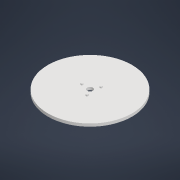
# Autodesk Inventor part: Carousel
Saved by Autodesk Inventor 2022 (Build 260153000, 153)
## iProperties
Created: 2021-10-09
Part Number: Carousel
Material: Generic
Document SubType Name: Modeling
Designer: zehrab
Density: 1 g/cm^3
Appearance: Default
Author: zehrab
Autodesk Inventor part; units mm, degrees
ref_plane "YZ Plane" through (0, 0, 0) normal (1, 0, 0) x (0, 1, 0)
ref_plane "XZ Plane" through (0, 0, 0) normal (0, 1, 0) x (-1, 0, 0)
ref_plane "XY Plane" through (0, 0, 0) normal (0, 0, 1) x (1, 0, 0)
sketch "Sketch1" plane through (0, 0, 0) normal (0, 1, 0) x (-1, 0, 0)
  circle A0 centre (0, 0) radius 12.7
  circle A1 centre (0, 0) radius 190.5
  dimension "d0" = 25.4
  dimension "d1" = 381
  constraints: 2 centre point, 2 coincident
  measures "d0" diameter of A0
  measures "d1" diameter of A1
extrude "Extrusion1" add sketch "Sketch1" along normal blind 12.7
sketch "Sketch2" plane through (0, 12.7, 0) normal (0, 1, 0) x (1, 0, 0)
  circle A0 centre (18.3309, -31.75) radius 4.7625
  circle A1 centre (-36.6617, 0) radius 4.7625
  circle A2 centre (18.3309, 31.75) radius 4.7625
  point P0 (0, 0)
  point P1 (0, 0)
  dimension "d5" = 9.525
  dimension "d6" = 9.525
  dimension "d7" = 9.525
  constraints: 3 centre point, 1 coincident
  measures "d5" diameter of A0
  measures "d6" diameter of A1
  measures "d7" diameter of A2
extrude "Extrusion2" add sketch "Sketch2" along normal blind 6.35
body "Solid1"
